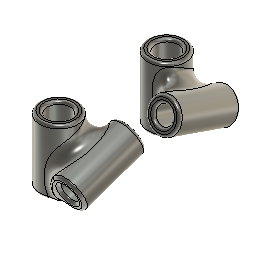
2-Attaches_base_V_avant (Autodesk Fusion 360 design; units mm, degrees)
Autodesk Fusion 360 part; units mm, degrees
sketch "Sketch1" plane through (0, 0, 0) normal (0, 0, 1) x (1, 0, 0)
  circle A0 centre (0, 0) radius 2.1
  circle A1 centre (0, 0) radius 3.5
  dimension "d1" = 4.2
  dimension "d2" = 7
  measures "d1" diameter of A0
  measures "d2" diameter of A1
extrude "Extrude1" add sketch "Sketch1" along normal blind 12 contours A1 picked at (3.012484, -0.278212) makes body 1
ref_plane "WorkPlane1" through (12.125, 0, 0) normal (0, 0.945519, 0.325568) x (1, 0, 0)
ref_plane "WorkPlane2" through (12.125, -2.836556, -0.976704) normal (0, 0.945519, 0.325568) x (1, 0, 0)
sketch "Sketch2" plane through (12.125, -2.836556, -0.976704) normal (0, 0.945519, 0.325568) x (1, 0, 0)
  circle A0 centre (-6, -5) radius 3
  circle A1 centre (-6, -5) radius 1.6
  dimension "d7" = 6
  dimension "d8" = 3.2
  measures "d7" diameter of A0
  measures "d8" diameter of A1
extrude "Extrude2" add sketch "Sketch2" along normal blind 12 contours A0 picked at (-3.483793, -5.228532) bodies 1
fillet "Fillet1" radius 2 1 edges at (3.5, 0, 6.824159) on bodies 1
fillet "Fillet2" radius 0.5 1 edges at (-3.263146, -1.265654, 12) on bodies 1
fillet "Fillet3" radius 0.5 1 edges at (-1.957887, 0.759392, 12) on bodies 1
fillet "Fillet4" radius 0.5 1 edges at (4.633276, -4.276028, 3.203826) on bodies 1
fillet "Fillet5" radius 0.5 2 edges at (2.898562, -3.758724, 1.701466) (8.89561, -4.838973, 4.838737) on bodies 1
fillet "Fillet6" radius 0.5 1 edges at (3.328018, 6.528635, 8.683449) on bodies 1
fillet "Fillet7" radius 0.5 1 edges at (4.633276, 7.070195, 7.110644) on bodies 1
fillet "Fillet8" radius 0.5 2 edges at (3.08989, -1.947563, 0) (-2.956367, 1.873471, 0) on bodies 1
fillet "Fillet9" radius 0.5 1 edges at (-1.957887, 0.759392, 0) on bodies 1
ref_plane "WorkPlane3" through (0, 10, 0) normal (0, 1, 0) x (0, 0, 1)
mirror "Mirror1" about plane through (0, 10, 0) normal (0, 1, 0) of bodies 1 makes body 2
